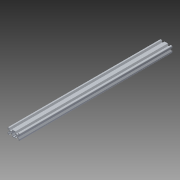
# Autodesk Inventor part: vslot_20x40x500
Saved by Autodesk Inventor 2015 (Build 190159000, 159)
## iProperties
Created: 2013-10-07
Part Number: vslot_20x40x500
Material: Generic
Document SubType Name: Modeling
Designer: Michael
Density: 1 g/cm^3
Appearance: Default
Sending System: SolidWorks 2011
Last Author: LAURENT Amaury
Author: Michael
Autodesk Inventor part; units mm, degrees
ref_plane "YZ Plane" through (0, 0, 0) normal (1, 0, 0) x (0, 1, 0)
ref_plane "XZ Plane" through (0, 0, 0) normal (0, 1, 0) x (-1, 0, 0)
ref_plane "Work Plane2" through (-5.36, -10, 250) normal (0, 0, 1) x (1, 0, 0)
sketch "Sketch1" plane through (-5.36, -10, 250) normal (0, 0, 1) x (1, 0, 0)
  line L0 (-1.8, 13.9007) -> (-7.48, 13.9007) projected
  line L1 (-7.48, 13.9007) -> (-10.1393, 16.56) projected
  line L2 (-10.1393, 16.56) -> (-10.1393, 18.2) projected
  line L3 (-10.1393, 18.2) -> (-7.48, 18.2) projected
  line L4 (-7.48, 18.2) -> (-9.28, 20) projected
  line L5 (-9.28, 20) -> (-12.84, 20) projected
  arc A0 (-12.84, 20) -> (-14.64, 18.2) centre (-12.84, 18.2) ccw projected
  line L6 (-14.64, 18.2) -> (-14.64, 14.64) projected
  line L7 (-14.64, 14.64) -> (-12.84, 12.84) projected
  line L8 (-12.84, 12.84) -> (-12.84, 15.4993) projected
  line L9 (-12.84, 15.4993) -> (-11.2, 15.4993) projected
  line L10 (-11.2, 15.4993) -> (-8.5407, 12.84) projected
  line L11 (-8.5407, 12.84) -> (-8.5407, 7.16) projected
  line L12 (-8.5407, 7.16) -> (-11.2, 4.5007) projected
  line L13 (-11.2, 4.5007) -> (-12.84, 4.5007) projected
  line L14 (-12.84, 4.5007) -> (-12.84, 7.16) projected
  line L15 (-12.84, 7.16) -> (-14.64, 5.36) projected
  line L16 (-14.64, 5.36) -> (-14.64, 1.8) projected
  arc A1 (-14.64, 1.8) -> (-12.84, 0) centre (-12.84, 1.8) ccw projected
  line L17 (-12.84, 0) -> (-9.28, 0) projected
  line L18 (-9.28, 0) -> (-7.48, 1.8) projected
  line L19 (-7.48, 1.8) -> (-10.1393, 1.8) projected
  line L20 (-10.1393, 1.8) -> (-10.1393, 3.44) projected
  line L21 (-10.1393, 3.44) -> (-7.48, 6.0993) projected
  line L22 (-7.48, 6.0993) -> (-1.8, 6.0993) projected
  line L23 (-1.8, 6.0993) -> (0.8593, 3.44) projected
  line L24 (0.8593, 3.44) -> (0.8593, 1.8) projected
  line L25 (0.8593, 1.8) -> (-1.8, 1.8) projected
  line L26 (-1.8, 1.8) -> (0, 0) projected
  line L27 (0, 0) -> (10.72, 0) projected
  line L28 (10.72, 0) -> (12.52, 1.8) projected
  line L29 (12.52, 1.8) -> (9.8607, 1.8) projected
  line L30 (9.8607, 1.8) -> (9.8607, 3.44) projected
  line L31 (9.8607, 3.44) -> (12.52, 6.0993) projected
  line L32 (12.52, 6.0993) -> (18.2, 6.0993) projected
  line L33 (18.2, 6.0993) -> (20.8593, 3.44) projected
  line L34 (20.8593, 3.44) -> (20.8593, 1.8) projected
  line L35 (20.8593, 1.8) -> (18.2, 1.8) projected
  line L36 (18.2, 1.8) -> (20, 0) projected
  line L37 (20, 0) -> (23.56, 0) projected
  arc A2 (23.56, 0) -> (25.36, 1.8) centre (23.56, 1.8) ccw projected
  line L38 (25.36, 1.8) -> (25.36, 5.36) projected
  line L39 (25.36, 5.36) -> (23.56, 7.16) projected
  line L40 (23.56, 7.16) -> (23.56, 4.5007) projected
  line L41 (23.56, 4.5007) -> (21.92, 4.5007) projected
  line L42 (21.92, 4.5007) -> (19.2607, 7.16) projected
  line L43 (19.2607, 7.16) -> (19.2607, 12.84) projected
  line L44 (19.2607, 12.84) -> (21.92, 15.4993) projected
  line L45 (21.92, 15.4993) -> (23.56, 15.4993) projected
  line L46 (23.56, 15.4993) -> (23.56, 12.84) projected
  line L47 (23.56, 12.84) -> (25.36, 14.64) projected
  line L48 (25.36, 14.64) -> (25.36, 18.2) projected
  arc A3 (25.36, 18.2) -> (23.56, 20) centre (23.56, 18.2) ccw projected
  line L49 (23.56, 20) -> (20, 20) projected
  line L50 (20, 20) -> (18.2, 18.2) projected
  line L51 (18.2, 18.2) -> (20.8593, 18.2) projected
  line L52 (20.8593, 18.2) -> (20.8593, 16.56) projected
  line L53 (20.8593, 16.56) -> (18.2, 13.9007) projected
  line L54 (18.2, 13.9007) -> (12.52, 13.9007) projected
  line L55 (12.52, 13.9007) -> (9.8607, 16.56) projected
  line L56 (9.8607, 16.56) -> (9.8607, 18.2) projected
  line L57 (9.8607, 18.2) -> (12.52, 18.2) projected
  line L58 (12.52, 18.2) -> (10.72, 20) projected
  line L59 (10.72, 20) -> (0, 20) projected
  line L60 (0, 20) -> (-1.8, 18.2) projected
  line L61 (-1.8, 18.2) -> (0.8593, 18.2) projected
  line L62 (0.8593, 18.2) -> (0.8593, 16.56) projected
  line L63 (0.8593, 16.56) -> (-1.8, 13.9007) projected
  circle A4 centre (-4.64, 10) radius 2.1 projected
  line L64 (-12.84, 1.8) -> (-11.2093, 1.8) projected
  line L65 (-12.84, 3.4307) -> (-12.84, 1.8) projected
  line L66 (-12.27, 3.4307) -> (-12.84, 3.4307) projected
  line L67 (-11.2093, 2.37) -> (-12.27, 3.4307) projected
  line L68 (-11.2093, 1.8) -> (-11.2093, 2.37) projected
  line L69 (23.56, 16.5693) -> (23.56, 18.2) projected
  line L70 (22.99, 16.5693) -> (23.56, 16.5693) projected
  line L71 (21.9293, 17.63) -> (22.99, 16.5693) projected
  line L72 (21.9293, 18.2) -> (21.9293, 17.63) projected
  line L73 (23.56, 18.2) -> (21.9293, 18.2) projected
  circle A5 centre (15.36, 10) radius 2.1 projected
  line L74 (23.56, 1.8) -> (23.56, 3.4307) projected
  line L75 (21.9293, 1.8) -> (23.56, 1.8) projected
  line L76 (21.9293, 2.37) -> (21.9293, 1.8) projected
  line L77 (22.99, 3.4307) -> (21.9293, 2.37) projected
  line L78 (23.56, 3.4307) -> (22.99, 3.4307) projected
  line L79 (-11.2093, 18.2) -> (-12.84, 18.2) projected
  line L80 (-11.2093, 17.63) -> (-11.2093, 18.2) projected
  line L81 (-12.27, 16.5693) -> (-11.2093, 17.63) projected
  line L82 (-12.84, 16.5693) -> (-12.27, 16.5693) projected
  line L83 (-12.84, 18.2) -> (-12.84, 16.5693) projected
  line L84 (8.06, 18.2) -> (2.66, 18.2) projected
  line L85 (8.06, 16.2393) -> (8.06, 18.2) projected
  line L86 (11.4593, 12.84) -> (8.06, 16.2393) projected
  line L87 (11.4593, 7.16) -> (11.4593, 12.84) projected
  line L88 (8.06, 3.7607) -> (11.4593, 7.16) projected
  line L89 (8.06, 1.8) -> (8.06, 3.7607) projected
  line L90 (2.66, 1.8) -> (8.06, 1.8) projected
  line L91 (2.66, 3.7607) -> (2.66, 1.8) projected
  line L92 (-0.7393, 7.16) -> (2.66, 3.7607) projected
  line L93 (-0.7393, 12.84) -> (-0.7393, 7.16) projected
  line L94 (2.66, 16.2393) -> (-0.7393, 12.84) projected
  line L95 (2.66, 18.2) -> (2.66, 16.2393) projected
  point P0 (5.36, 10)
extrude "Extrusion2" add sketch "Sketch1" against normal blind 500
body "Solid3"
